Autodesk Fusion 360 part; units mm, degrees
(part 3 of 5)
  spline S32 degree 5 poles (-178.9509, -27.9451) (-178.953, -27.9386) (-178.9574, -27.9258) (-178.9646, -27.9067) (-178.975, -27.8817) (-178.9895, -27.8509) (-179.005, -27.8206) (-179.021, -27.7904) (-179.0374, -27.7604) (-179.0541, -27.7304) (-179.0709, -27.7005) (-179.0881, -27.6708) (-179.1057, -27.6412) (-179.1237, -27.6118) (-179.1422, -27.5825) (-179.1612, -27.5535) (-179.1805, -27.5247) (-179.2001, -27.4959) (-179.22, -27.4673) (-179.2402, -27.4388) (-179.2607, -27.4105) (-179.2814, -27.3822) (-179.3023, -27.3541) (-179.3236, -27.3261) (-179.3452, -27.2982) (-179.367, -27.2705) (-179.3891, -27.2429) (-179.4115, -27.2154) (-179.4341, -27.188) (-179.457, -27.1608) (-179.48, -27.1336) (-179.5033, -27.1066) (-179.5269, -27.0797) (-179.5506, -27.0529) (-179.5746, -27.0263) (-179.5989, -26.9997) (-179.6233, -26.9733) (-179.648, -26.947) (-179.6728, -26.9208) (-179.6979, -26.8947) (-179.7232, -26.8687) (-179.7487, -26.8428) (-179.7744, -26.8171) (-179.8003, -26.7914) (-179.8264, -26.7659) (-179.8527, -26.7405) (-179.8792, -26.7152) (-179.9058, -26.69) (-179.9327, -26.6649) (-179.9598, -26.64) (-179.987, -26.6151) (-180.0144, -26.5904) (-180.0421, -26.5658) (-180.0699, -26.5412) (-180.0978, -26.5168) (-180.126, -26.4926) (-180.1543, -26.4684) (-180.1828, -26.4443) (-180.2115, -26.4204) (-180.2404, -26.3965) (-180.2694, -26.3728) (-180.2986, -26.3492) (-180.3279, -26.3257) (-180.3575, -26.3023) (-180.3872, -26.279) (-180.417, -26.2558) (-180.447, -26.2328) (-180.4772, -26.2099) (-180.5076, -26.187) (-180.5381, -26.1643) (-180.5687, -26.1417) (-180.5934, -26.1237) (-180.612, -26.1103) (-180.6244, -26.1014) (-180.6306, -26.0969) knots 0 0 0 0 0 0 0.01428571 0.02857143 0.04285714 0.05714286 0.07142857 0.08571429 0.1 0.11428571 0.12857143 0.14285714 0.15714286 0.17142857 0.18571429 0.2 0.21428571 0.22857143 0.24285714 0.25714286 0.27142857 0.28571429 0.3 0.31428571 0.32857143 0.34285714 0.35714286 0.37142857 0.38571429 0.4 0.41428571 0.42857143 0.44285714 0.45714286 0.47142857 0.48571429 0.5 0.51428571 0.52857143 0.54285714 0.55714286 0.57142857 0.58571429 0.6 0.61428571 0.62857143 0.64285714 0.65714286 0.67142857 0.68571429 0.7 0.71428571 0.72857143 0.74285714 0.75714286 0.77142857 0.78571429 0.8 0.81428571 0.82857143 0.84285714 0.85714286 0.87142857 0.88571429 0.9 0.91428571 0.92857143 0.94285714 0.95714286 0.97142857 0.98571429 1 1 1 1 1 1
  arc A65 (-180.6306, -26.0969) -> (-181.4895, -26.4764) centre (-175, -40) ccw
  spline S33 degree 5 poles (-181.2537, -28.9627) (-181.2571, -28.9568) (-181.2636, -28.9449) (-181.2729, -28.9268) (-181.2843, -28.9022) (-181.2973, -28.8708) (-181.3094, -28.8389) (-181.3209, -28.8067) (-181.332, -28.7744) (-181.343, -28.7419) (-181.3537, -28.7093) (-181.3642, -28.6766) (-181.3743, -28.6437) (-181.3839, -28.6105) (-181.393, -28.5772) (-181.4017, -28.5436) (-181.41, -28.5099) (-181.418, -28.476) (-181.4258, -28.4421) (-181.4333, -28.408) (-181.4405, -28.3737) (-181.4474, -28.3394) (-181.4541, -28.305) (-181.4605, -28.2704) (-181.4666, -28.2357) (-181.4724, -28.2008) (-181.4779, -28.1659) (-181.4832, -28.1309) (-181.4882, -28.0957) (-181.493, -28.0605) (-181.4975, -28.0252) (-181.5018, -27.9897) (-181.5058, -27.9542) (-181.5096, -27.9186) (-181.5132, -27.8829) (-181.5165, -27.8471) (-181.5196, -27.8113) (-181.5225, -27.7753) (-181.5251, -27.7393) (-181.5275, -27.7032) (-181.5297, -27.667) (-181.5316, -27.6307) (-181.5334, -27.5944) (-181.5349, -27.558) (-181.5362, -27.5215) (-181.5373, -27.4849) (-181.5382, -27.4483) (-181.5388, -27.4116) (-181.5393, -27.3749) (-181.5395, -27.3381) (-181.5396, -27.3012) (-181.5394, -27.2643) (-181.539, -27.2273) (-181.5384, -27.1902) (-181.5376, -27.1531) (-181.5366, -27.1159) (-181.5354, -27.0787) (-181.534, -27.0414) (-181.5324, -27.0041) (-181.5306, -26.9667) (-181.5286, -26.9293) (-181.5264, -26.8918) (-181.524, -26.8542) (-181.5215, -26.8167) (-181.5187, -26.779) (-181.5157, -26.7414) (-181.5125, -26.7036) (-181.5092, -26.6659) (-181.5056, -26.6281) (-181.5019, -26.5902) (-181.4979, -26.5523) (-181.4947, -26.522) (-181.4921, -26.4992) (-181.4903, -26.484) (-181.4895, -26.4764) knots 0 0 0 0 0 0 0.01428571 0.02857143 0.04285714 0.05714286 0.07142857 0.08571429 0.1 0.11428571 0.12857143 0.14285714 0.15714286 0.17142857 0.18571429 0.2 0.21428571 0.22857143 0.24285714 0.25714286 0.27142857 0.28571429 0.3 0.31428571 0.32857143 0.34285714 0.35714286 0.37142857 0.38571429 0.4 0.41428571 0.42857143 0.44285714 0.45714286 0.47142857 0.48571429 0.5 0.51428571 0.52857143 0.54285714 0.55714286 0.57142857 0.58571429 0.6 0.61428571 0.62857143 0.64285714 0.65714286 0.67142857 0.68571429 0.7 0.71428571 0.72857143 0.74285714 0.75714286 0.77142857 0.78571429 0.8 0.81428571 0.82857143 0.84285714 0.85714286 0.87142857 0.88571429 0.9 0.91428571 0.92857143 0.94285714 0.95714286 0.97142857 0.98571429 1 1 1 1 1 1
  line L33 (-181.2537, -28.9627) -> (-181.041, -29.3382)
  arc A66 (-181.212, -30.0093) -> (-181.041, -29.3382) centre (-181.476, -29.5847) ccw
  arc A67 (-181.212, -30.0093) -> (-181.8833, -30.4594) centre (-175, -40) ccw
  arc A68 (-182.5691, -30.3628) -> (-181.8833, -30.4594) centre (-182.1759, -30.0539) ccw
  line L34 (-182.5691, -30.3628) -> (-182.8357, -30.0234)
  spline S34 degree 5 poles (-182.8357, -30.0234) (-182.8399, -30.018) (-182.8484, -30.0075) (-182.8616, -29.992) (-182.88, -29.9721) (-182.9041, -29.9481) (-182.9291, -29.9248) (-182.9545, -29.902) (-182.9801, -29.8794) (-183.006, -29.8569) (-183.0321, -29.8346) (-183.0584, -29.8125) (-183.085, -29.7907) (-183.112, -29.7692) (-183.1394, -29.7481) (-183.1671, -29.7273) (-183.1952, -29.7068) (-183.2235, -29.6866) (-183.252, -29.6665) (-183.2807, -29.6466) (-183.3096, -29.6269) (-183.3387, -29.6075) (-183.368, -29.5882) (-183.3976, -29.5692) (-183.4274, -29.5504) (-183.4574, -29.5318) (-183.4876, -29.5134) (-183.5181, -29.4952) (-183.5487, -29.4772) (-183.5794, -29.4594) (-183.6104, -29.4418) (-183.6415, -29.4244) (-183.6729, -29.4072) (-183.7044, -29.3901) (-183.736, -29.3733) (-183.7679, -29.3566) (-183.7999, -29.3401) (-183.8321, -29.3238) (-183.8644, -29.3077) (-183.8969, -29.2918) (-183.9295, -29.276) (-183.9623, -29.2604) (-183.9953, -29.245) (-184.0284, -29.2298) (-184.0616, -29.2147) (-184.095, -29.1999) (-184.1286, -29.1851) (-184.1623, -29.1706) (-184.1961, -29.1562) (-184.2301, -29.142) (-184.2642, -29.128) (-184.2984, -29.1141) (-184.3328, -29.1004) (-184.3673, -29.0869) (-184.4019, -29.0735) (-184.4367, -29.0603) (-184.4716, -29.0473) (-184.5066, -29.0345) (-184.5417, -29.0218) (-184.577, -29.0092) (-184.6124, -28.9969) (-184.6479, -28.9847) (-184.6835, -28.9726) (-184.7193, -28.9607) (-184.7551, -28.949) (-184.7911, -28.9375) (-184.8272, -28.9261) (-184.8634, -28.9148) (-184.8997, -28.9038) (-184.9362, -28.8928) (-184.9727, -28.8821) (-185.002, -28.8736) (-185.0241, -28.8673) (-185.0388, -28.8632) (-185.0462, -28.8611) knots 0 0 0 0 0 0 0.01428571 0.02857143 0.04285714 0.05714286 0.07142857 0.08571429 0.1 0.11428571 0.12857143 0.14285714 0.15714286 0.17142857 0.18571429 0.2 0.21428571 0.22857143 0.24285714 0.25714286 0.27142857 0.28571429 0.3 0.31428571 0.32857143 0.34285714 0.35714286 0.37142857 0.38571429 0.4 0.41428571 0.42857143 0.44285714 0.45714286 0.47142857 0.48571429 0.5 0.51428571 0.52857143 0.54285714 0.55714286 0.57142857 0.58571429 0.6 0.61428571 0.62857143 0.64285714 0.65714286 0.67142857 0.68571429 0.7 0.71428571 0.72857143 0.74285714 0.75714286 0.77142857 0.78571429 0.8 0.81428571 0.82857143 0.84285714 0.85714286 0.87142857 0.88571429 0.9 0.91428571 0.92857143 0.94285714 0.95714286 0.97142857 0.98571429 1 1 1 1 1 1
  arc A69 (-185.0462, -28.8611) -> (-185.7234, -29.5115) centre (-175, -40) ccw
  spline S35 degree 5 poles (-184.6515, -31.7672) (-184.6567, -31.7628) (-184.6669, -31.7539) (-184.6818, -31.74) (-184.701, -31.7208) (-184.724, -31.6958) (-184.7462, -31.6699) (-184.768, -31.6436) (-184.7896, -31.617) (-184.811, -31.5903) (-184.8322, -31.5633) (-184.8532, -31.5362) (-184.8739, -31.5087) (-184.8943, -31.4808) (-184.9143, -31.4526) (-184.9339, -31.424) (-184.9533, -31.3952) (-184.9724, -31.3661) (-184.9913, -31.3368) (-185.01, -31.3073) (-185.0285, -31.2777) (-185.0468, -31.2478) (-185.0648, -31.2177) (-185.0826, -31.1874) (-185.1002, -31.1568) (-185.1176, -31.1261) (-185.1347, -31.0952) (-185.1517, -31.064) (-185.1684, -31.0327) (-185.1849, -31.0013) (-185.2013, -30.9696) (-185.2174, -30.9378) (-185.2334, -30.9058) (-185.2491, -30.8736) (-185.2647, -30.8413) (-185.28, -30.8088) (-185.2952, -30.7762) (-185.3102, -30.7434) (-185.325, -30.7104) (-185.3396, -30.6773) (-185.354, -30.644) (-185.3683, -30.6106) (-185.3823, -30.5771) (-185.3962, -30.5434) (-185.4099, -30.5096) (-185.4235, -30.4756) (-185.4368, -30.4415) (-185.45, -30.4072) (-185.463, -30.3728) (-185.4758, -30.3383) (-185.4884, -30.3037) (-185.5009, -30.2689) (-185.5132, -30.234) (-185.5253, -30.199) (-185.5372, -30.1639) (-185.549, -30.1286) (-185.5606, -30.0932) (-185.5721, -30.0577) (-185.5833, -30.0221) (-185.5944, -29.9863) (-185.6054, -29.9505) (-185.6161, -29.9145) (-185.6267, -29.8784) (-185.6371, -29.8422) (-185.6474, -29.8059) (-185.6575, -29.7695) (-185.6674, -29.7329) (-185.6772, -29.6963) (-185.6868, -29.6596) (-185.6962, -29.6227) (-185.7054, -29.5858) (-185.7127, -29.5561) (-185.7181, -29.5338) (-185.7217, -29.519) (-185.7234, -29.5115) knots 0 0 0 0 0 0 0.01428571 0.02857143 0.04285714 0.05714286 0.07142857 0.08571429 0.1 0.11428571 0.12857143 0.14285714 0.15714286 0.17142857 0.18571429 0.2 0.21428571 0.22857143 0.24285714 0.25714286 0.27142857 0.28571429 0.3 0.31428571 0.32857143 0.34285714 0.35714286 0.37142857 0.38571429 0.4 0.41428571 0.42857143 0.44285714 0.45714286 0.47142857 0.48571429 0.5 0.51428571 0.52857143 0.54285714 0.55714286 0.57142857 0.58571429 0.6 0.61428571 0.62857143 0.64285714 0.65714286 0.67142857 0.68571429 0.7 0.71428571 0.72857143 0.74285714 0.75714286 0.77142857 0.78571429 0.8 0.81428571 0.82857143 0.84285714 0.85714286 0.87142857 0.88571429 0.9 0.91428571 0.92857143 0.94285714 0.95714286 0.97142857 0.98571429 1 1 1 1 1 1
  line L35 (-184.6515, -31.7672) -> (-184.3232, -32.0473)
  arc A70 (-184.2544, -32.7364) -> (-184.3232, -32.0473) centre (-184.6477, -32.4277) ccw
  arc A71 (-184.2544, -32.7364) -> (-184.7313, -33.389) centre (-175, -40) ccw
  circle A72 centre (-175, -40) radius 4
  line L36 (250, 25) -> (120, 25)
  line L37 (120, 25) -> (120, 175)
  line L38 (120, 175) -> (250, 175)
  line L39 (250, 175) -> (250, 25)
  dimension "d74" = 130
  dimension "d75" = 150
  constraint horizontal L36
  constraint vertical L37
  constraint horizontal L38
  constraint vertical L39
  measures "d74" distance of L36.start L36.end
  measures "d75" distance of L36.start L38.end
extrude "Extrude4" add sketch "SamsungFold4DeschisHusa" along normal blind 10 separate body contours L36 L37 L38 L39 makes body 5
sketch "Sketch6" plane through (0, 10, 0) normal (0, 1, 0) x (-1, 0, 0)
  arc A0 (-122.7744, -52.0505) -> (-123.3367, -51.6463) centre (-123.266, -52.1413) ccw
  line L0 (-122.7744, -52.0505) -> (-122.696, -52.4749)
  spline S0 degree 5 poles (-122.696, -52.4749) (-122.6947, -52.4815) (-122.6921, -52.4949) (-122.6876, -52.5147) (-122.6805, -52.5409) (-122.6703, -52.5733) (-122.6591, -52.6055) (-122.6472, -52.6375) (-122.6349, -52.6695) (-122.6225, -52.7014) (-122.6097, -52.7333) (-122.5967, -52.7651) (-122.5833, -52.7967) (-122.5693, -52.8283) (-122.5549, -52.8597) (-122.54, -52.891) (-122.5247, -52.9222) (-122.509, -52.9533) (-122.4931, -52.9843) (-122.4769, -53.0152) (-122.4605, -53.0461) (-122.4437, -53.0769) (-122.4267, -53.1076) (-122.4094, -53.1381) (-122.3917, -53.1686) (-122.3738, -53.199) (-122.3555, -53.2293) (-122.3371, -53.2596) (-122.3183, -53.2897) (-122.2993, -53.3198) (-122.2801, -53.3498) (-122.2606, -53.3797) (-122.2409, -53.4095) (-122.2209, -53.4392) (-122.2007, -53.4688) (-122.1802, -53.4984) (-122.1595, -53.5278) (-122.1386, -53.5572) (-122.1175, -53.5865) (-122.0961, -53.6157) (-122.0745, -53.6448) (-122.0527, -53.6739) (-122.0307, -53.7028) (-122.0085, -53.7317) (-121.986, -53.7605) (-121.9633, -53.7892) (-121.9405, -53.8178) (-121.9174, -53.8463) (-121.8941, -53.8748) (-121.8706, -53.9031) (-121.847, -53.9314) (-121.8231, -53.9596) (-121.799, -53.9877) (-121.7747, -54.0157) (-121.7503, -54.0436) (-121.7256, -54.0714) (-121.7008, -54.0992) (-121.6757, -54.1268) (-121.6505, -54.1544) (-121.6251, -54.1819) (-121.5995, -54.2093) (-121.5737, -54.2366) (-121.5478, -54.2638) (-121.5216, -54.2909) (-121.4953, -54.318) (-121.4688, -54.3449) (-121.4422, -54.3718) (-121.4153, -54.3985) (-121.3883, -54.4252) (-121.3611, -54.4518) (-121.3337, -54.4783) (-121.3117, -54.4994) (-121.2951, -54.5152) (-121.284, -54.5257) (-121.2784, -54.531) knots 0 0 0 0 0 0 0.01428571 0.02857143 0.04285714 0.05714286 0.07142857 0.08571429 0.1 0.11428571 0.12857143 0.14285714 0.15714286 0.17142857 0.18571429 0.2 0.21428571 0.22857143 0.24285714 0.25714286 0.27142857 0.28571429 0.3 0.31428571 0.32857143 0.34285714 0.35714286 0.37142857 0.38571429 0.4 0.41428571 0.42857143 0.44285714 0.45714286 0.47142857 0.48571429 0.5 0.51428571 0.52857143 0.54285714 0.55714286 0.57142857 0.58571429 0.6 0.61428571 0.62857143 0.64285714 0.65714286 0.67142857 0.68571429 0.7 0.71428571 0.72857143 0.74285714 0.75714286 0.77142857 0.78571429 0.8 0.81428571 0.82857143 0.84285714 0.85714286 0.87142857 0.88571429 0.9 0.91428571 0.92857143 0.94285714 0.95714286 0.97142857 0.98571429 1 1 1 1 1 1
  arc A1 (-121.2784, -54.531) -> (-120.3765, -54.2697) centre (-125, -40) ccw
  spline S1 degree 5 poles (-120.2778, -51.7742) (-120.2753, -51.7805) (-120.2704, -51.7932) (-120.2636, -51.8124) (-120.2556, -51.8383) (-120.2469, -51.8711) (-120.2392, -51.9043) (-120.2321, -51.9378) (-120.2254, -51.9713) (-120.2188, -52.005) (-120.2126, -52.0387) (-120.2066, -52.0725) (-120.201, -52.1065) (-120.1959, -52.1406) (-120.1913, -52.1749) (-120.1872, -52.2093) (-120.1834, -52.2438) (-120.18, -52.2785) (-120.1769, -52.3132) (-120.174, -52.348) (-120.1714, -52.3828) (-120.1691, -52.4178) (-120.1671, -52.4528) (-120.1654, -52.488) (-120.1641, -52.5232) (-120.163, -52.5585) (-120.1622, -52.5938) (-120.1616, -52.6292) (-120.1613, -52.6647) (-120.1613, -52.7003) (-120.1616, -52.7359) (-120.162, -52.7716) (-120.1628, -52.8073) (-120.1638, -52.8431) (-120.165, -52.879) (-120.1665, -52.9149) (-120.1682, -52.9508) (-120.1702, -52.9869) (-120.1724, -53.0229) (-120.1749, -53.059) (-120.1775, -53.0952) (-120.1804, -53.1314) (-120.1836, -53.1676) (-120.1869, -53.2039) (-120.1905, -53.2402) (-120.1943, -53.2766) (-120.1983, -53.313) (-120.2026, -53.3495) (-120.2071, -53.3859) (-120.2117, -53.4224) (-120.2166, -53.459) (-120.2218, -53.4956) (-120.2271, -53.5322) (-120.2326, -53.5688) (-120.2384, -53.6055) (-120.2443, -53.6422) (-120.2505, -53.679) (-120.2569, -53.7157) (-120.2634, -53.7525) (-120.2702, -53.7893) (-120.2772, -53.8261) (-120.2844, -53.863) (-120.2918, -53.8999) (-120.2993, -53.9368) (-120.3071, -53.9737) (-120.3151, -54.0106) (-120.3233, -54.0476) (-120.3317, -54.0846) (-120.3402, -54.1215) (-120.349, -54.1586) (-120.358, -54.1956) (-120.3653, -54.2252) (-120.3709, -54.2474) (-120.3746, -54.2623) (-120.3765, -54.2697) knots 0 0 0 0 0 0 0.01428571 0.02857143 0.04285714 0.05714286 0.07142857 0.08571429 0.1 0.11428571 0.12857143 0.14285714 0.15714286 0.17142857 0.18571429 0.2 0.21428571 0.22857143 0.24285714 0.25714286 0.27142857 0.28571429 0.3 0.31428571 0.32857143 0.34285714 0.35714286 0.37142857 0.38571429 0.4 0.41428571 0.42857143 0.44285714 0.45714286 0.47142857 0.48571429 0.5 0.51428571 0.52857143 0.54285714 0.55714286 0.57142857 0.58571429 0.6 0.61428571 0.62857143 0.64285714 0.65714286 0.67142857 0.68571429 0.7 0.71428571 0.72857143 0.74285714 0.75714286 0.77142857 0.78571429 0.8 0.81428571 0.82857143 0.84285714 0.85714286 0.87142857 0.88571429 0.9 0.91428571 0.92857143 0.94285714 0.95714286 0.97142857 0.98571429 1 1 1 1 1 1
  line L1 (-120.2778, -51.7742) -> (-120.4385, -51.3737)
  arc A2 (-120.1793, -50.7315) -> (-120.4385, -51.3737) centre (-119.9744, -51.1875) ccw
  arc A3 (-120.1793, -50.7315) -> (-119.4538, -50.3751) centre (-125, -40) ccw
  arc A4 (-118.7871, -50.5625) -> (-119.4538, -50.3751) centre (-119.218, -50.816) ccw
  line L2 (-118.7871, -50.5625) -> (-118.5683, -50.9345)
  spline S2 degree 5 poles (-118.5683, -50.9345) (-118.5648, -50.9404) (-118.5578, -50.952) (-118.5468, -50.9691) (-118.5312, -50.9913) (-118.5105, -51.0183) (-118.4889, -51.0446) (-118.4668, -51.0707) (-118.4443, -51.0965) (-118.4217, -51.1223) (-118.3989, -51.1478) (-118.3757, -51.1733) (-118.3523, -51.1984) (-118.3284, -51.2233) (-118.304, -51.2479) (-118.2793, -51.2722) (-118.2543, -51.2963) (-118.229, -51.3202) (-118.2034, -51.3439) (-118.1776, -51.3674) (-118.1516, -51.3908) (-118.1254, -51.4139) (-118.0989, -51.437) (-118.0721, -51.4598) (-118.0451, -51.4824) (-118.0178, -51.5048) (-117.9903, -51.5271) (-117.9626, -51.5491) (-117.9347, -51.5711) (-117.9066, -51.5928) (-117.8782, -51.6144) (-117.8497, -51.6358) (-117.821, -51.6571) (-117.792, -51.6782) (-117.7629, -51.6991) (-117.7336, -51.7199) (-117.704, -51.7405) (-117.6743, -51.761) (-117.6445, -51.7813) (-117.6144, -51.8014) (-117.5841, -51.8214) (-117.5537, -51.8412) (-117.5231, -51.8609) (-117.4923, -51.8804) (-117.4614, -51.8998) (-117.4303, -51.919) (-117.399, -51.9381) (-117.3676, -51.957) (-117.336, -51.9757) (-117.3042, -51.9944) (-117.2723, -52.0128) (-117.2402, -52.0311) (-117.208, -52.0493) (-117.1756, -52.0673) (-117.1431, -52.0852) (-117.1104, -52.1029) (-117.0775, -52.1205) (-117.0446, -52.1379) (-117.0114, -52.1552) (-116.9781, -52.1723) (-116.9447, -52.1893) (-116.9112, -52.2062) (-116.8775, -52.2229) (-116.8436, -52.2394) (-116.8096, -52.2558) (-116.7755, -52.2721) (-116.7413, -52.2882) (-116.7069, -52.3042) (-116.6724, -52.32) (-116.6377, -52.3357) (-116.603, -52.3512) (-116.575, -52.3635) (-116.554, -52.3727) (-116.54, -52.3788) (-116.533, -52.3818) knots 0 0 0 0 0 0 0.01428571 0.02857143 0.04285714 0.05714286 0.07142857 0.08571429 0.1 0.11428571 0.12857143 0.14285714 0.15714286 0.17142857 0.18571429 0.2 0.21428571 0.22857143 0.24285714 0.25714286 0.27142857 0.28571429 0.3 0.31428571 0.32857143 0.34285714 0.35714286 0.37142857 0.38571429 0.4 0.41428571 0.42857143 0.44285714 0.45714286 0.47142857 0.48571429 0.5 0.51428571 0.52857143 0.54285714 0.55714286 0.57142857 0.58571429 0.6 0.61428571 0.62857143 0.64285714 0.65714286 0.67142857 0.68571429 0.7 0.71428571 0.72857143 0.74285714 0.75714286 0.77142857 0.78571429 0.8 0.81428571 0.82857143 0.84285714 0.85714286 0.87142857 0.88571429 0.9 0.91428571 0.92857143 0.94285714 0.95714286 0.97142857 0.98571429 1 1 1 1 1 1
  arc A5 (-116.533, -52.3818) -> (-115.7748, -51.8278) centre (-125, -40) ccw
  spline S3 degree 5 poles (-116.5356, -49.4491) (-116.5311, -49.4541) (-116.5221, -49.4643) (-116.5092, -49.48) (-116.4928, -49.5016) (-116.4734, -49.5296) (-116.4548, -49.5581) (-116.4367, -49.5871) (-116.4189, -49.6163) (-116.4012, -49.6457) (-116.3838, -49.6753) (-116.3666, -49.705) (-116.3498, -49.735) (-116.3333, -49.7653) (-116.3173, -49.796) (-116.3016, -49.8269) (-116.2863, -49.8581) (-116.2712, -49.8894) (-116.2564, -49.921) (-116.2418, -49.9527) (-116.2275, -49.9846) (-116.2133, -50.0167) (-116.1995, -50.0489) (-116.1859, -50.0813) (-116.1725, -50.1139) (-116.1594, -50.1467) (-116.1466, -50.1797) (-116.134, -50.2128) (-116.1216, -50.246) (-116.1094, -50.2794) (-116.0974, -50.313) (-116.0857, -50.3467) (-116.0741, -50.3805) (-116.0628, -50.4145) (-116.0517, -50.4486) (-116.0408, -50.4829) (-116.0302, -50.5173) (-116.0197, -50.5518) (-116.0095, -50.5864) (-115.9994, -50.6212) (-115.9895, -50.6561) (-115.9799, -50.6911) (-115.9704, -50.7262) (-115.9612, -50.7614) (-115.9521, -50.7968) (-115.9433, -50.8323) (-115.9346, -50.8679) (-115.9261, -50.9036) (-115.9178, -50.9394) (-115.9098, -50.9753) (-115.9019, -51.0113) (-115.8942, -51.0474) (-115.8866, -51.0837) (-115.8793, -51.12) (-115.8722, -51.1564) (-115.8652, -51.193) (-115.8584, -51.2296) (-115.8518, -51.2663) (-115.8454, -51.3031) (-115.8392, -51.34) (-115.8332, -51.377) (-115.8273, -51.4141) (-115.8217, -51.4513) (-115.8162, -51.4886) (-115.8109, -51.5259) (-115.8057, -51.5634) (-115.8008, -51.6009) (-115.796, -51.6385) (-115.7914, -51.6762) (-115.787, -51.714) (-115.7827, -51.7518) (-115.7795, -51.7822) (-115.7771, -51.805) (-115.7756, -51.8202) (-115.7748, -51.8278) knots 0 0 0 0 0 0 0.01428571 0.02857143 0.04285714 0.05714286 0.07142857 0.08571429 0.1 0.11428571 0.12857143 0.14285714 0.15714286 0.17142857 0.18571429 0.2 0.21428571 0.22857143 0.24285714 0.25714286 0.27142857 0.28571429 0.3 0.31428571 0.32857143 0.34285714 0.35714286 0.37142857 0.38571429 0.4 0.41428571 0.42857143 0.44285714 0.45714286 0.47142857 0.48571429 0.5 0.51428571 0.52857143 0.54285714 0.55714286 0.57142857 0.58571429 0.6 0.61428571 0.62857143 0.64285714 0.65714286 0.67142857 0.68571429 0.7 0.71428571 0.72857143 0.74285714 0.75714286 0.77142857 0.78571429 0.8 0.81428571 0.82857143 0.84285714 0.85714286 0.87142857 0.88571429 0.9 0.91428571 0.92857143 0.94285714 0.95714286 0.97142857 0.98571429 1 1 1 1 1 1
  line L3 (-116.5356, -49.4491) -> (-116.8235, -49.1276)
  arc A6 (-116.7996, -48.4355) -> (-116.8235, -49.1276) centre (-116.4511, -48.794) ccw
  arc A7 (-116.7996, -48.4355) -> (-116.2397, -47.8525) centre (-125, -40) ccw
  arc A8 (-115.5491, -47.8006) -> (-116.2397, -47.8525) centre (-115.8674, -48.1862) ccw
  line L4 (-115.5491, -47.8006) -> (-115.2163, -48.0753)
  spline S4 degree 5 poles (-115.2163, -48.0753) (-115.2111, -48.0796) (-115.2005, -48.0881) (-115.1843, -48.1004) (-115.162, -48.116) (-115.1334, -48.1342) (-115.1041, -48.1516) (-115.0744, -48.1685) (-115.0445, -48.1852) (-115.0144, -48.2016) (-114.9842, -48.2178) (-114.9537, -48.2338) (-114.9231, -48.2494) (-114.8921, -48.2646) (-114.8609, -48.2794) (-114.8293, -48.2938) (-114.7976, -48.3079) (-114.7656, -48.3216) (-114.7335, -48.3352) (-114.7012, -48.3485) (-114.6687, -48.3615) (-114.6361, -48.3743) (-114.6034, -48.3869) (-114.5704, -48.3992) (-114.5373, -48.4112) (-114.504, -48.4229) (-114.4706, -48.4344) (-114.437, -48.4457) (-114.4032, -48.4568) (-114.3694, -48.4676) (-114.3354, -48.4782) (-114.3012, -48.4886) (-114.267, -48.4987) (-114.2325, -48.5086) (-114.198, -48.5183) (-114.1633, -48.5278) (-114.1286, -48.5371) (-114.0936, -48.5462) (-114.0586, -48.555) (-114.0235, -48.5637) (-113.9882, -48.5721) (-113.9528, -48.5803) (-113.9174, -48.5883) (-113.8818, -48.5962) (-113.8461, -48.6038) (-113.8103, -48.6112) (-113.7744, -48.6184) (-113.7383, -48.6254) (-113.7022, -48.6323) (-113.666, -48.6389) (-113.6297, -48.6453) (-113.5933, -48.6516) (-113.5568, -48.6576) (-113.5202, -48.6635) (-113.4835, -48.6691) (-113.4467, -48.6746) (-113.4099, -48.6799) (-113.3729, -48.685) (-113.3359, -48.6899) (-113.2987, -48.6946) (-113.2615, -48.6992) (-113.2242, -48.7035) (-113.1869, -48.7077) (-113.1494, -48.7116) (-113.1119, -48.7154) (-113.0742, -48.7191) (-113.0365, -48.7225) (-112.9988, -48.7257) (-112.9609, -48.7288) (-112.923, -48.7317) (-112.885, -48.7344) (-112.8545, -48.7364) (-112.8317, -48.7378) (-112.8164, -48.7388) (-112.8088, -48.7392) knots 0 0 0 0 0 0 0.01428571 0.02857143 0.04285714 0.05714286 0.07142857 0.08571429 0.1 0.11428571 0.12857143 0.14285714 0.15714286 0.17142857 0.18571429 0.2 0.21428571 0.22857143 0.24285714 0.25714286 0.27142857 0.28571429 0.3 0.31428571 0.32857143 0.34285714 0.35714286 0.37142857 0.38571429 0.4 0.41428571 0.42857143 0.44285714 0.45714286 0.47142857 0.48571429 0.5 0.51428571 0.52857143 0.54285714 0.55714286 0.57142857 0.58571429 0.6 0.61428571 0.62857143 0.64285714 0.65714286 0.67142857 0.68571429 0.7 0.71428571 0.72857143 0.74285714 0.75714286 0.77142857 0.78571429 0.8 0.81428571 0.82857143 0.84285714 0.85714286 0.87142857 0.88571429 0.9 0.91428571 0.92857143 0.94285714 0.95714286 0.97142857 0.98571429 1 1 1 1 1 1
  arc A9 (-112.8088, -48.7392) -> (-112.2858, -47.9593) centre (-125, -40) ccw
  spline S5 degree 5 poles (-113.8143, -45.9842) (-113.8083, -45.9874) (-113.7964, -45.994) (-113.7789, -46.0043) (-113.7561, -46.019) (-113.7283, -46.0386) (-113.701, -46.0591) (-113.6741, -46.0801) (-113.6474, -46.1015) (-113.6208, -46.1231) (-113.5943, -46.1449) (-113.568, -46.1669) (-113.5419, -46.1894) (-113.516, -46.2122) (-113.4905, -46.2355) (-113.4652, -46.2592) (-113.4401, -46.2833) (-113.4152, -46.3076) (-113.3905, -46.3322) (-113.366, -46.357) (-113.3416, -46.3821) (-113.3173, -46.4074) (-113.2933, -46.4329) (-113.2694, -46.4587) (-113.2457, -46.4848) (-113.2222, -46.5111) (-113.1989, -46.5377) (-113.1757, -46.5645) (-113.1526, -46.5915) (-113.1298, -46.6187) (-113.1071, -46.6462) (-113.0845, -46.6738) (-113.0621, -46.7017) (-113.0398, -46.7297) (-113.0177, -46.758) (-112.9958, -46.7865) (-112.974, -46.8151) (-112.9524, -46.844) (-112.9309, -46.873) (-112.9095, -46.9023) (-112.8884, -46.9317) (-112.8673, -46.9613) (-112.8464, -46.991) (-112.8257, -47.021) (-112.8051, -47.0511) (-112.7846, -47.0814) (-112.7643, -47.1119) (-112.7441, -47.1426) (-112.7241, -47.1734) (-112.7042, -47.2044) (-112.6845, -47.2355) (-112.6649, -47.2668) (-112.6454, -47.2983) (-112.6261, -47.3299) (-112.6069, -47.3617) (-112.5879, -47.3937) (-112.569, -47.4258) (-112.5502, -47.458) (-112.5316, -47.4904) (-112.5132, -47.523) (-112.4948, -47.5557) (-112.4767, -47.5885) (-112.4586, -47.6215) (-112.4407, -47.6547) (-112.4229, -47.6879) (-112.4053, -47.7214) (-112.3878, -47.7549) (-112.3705, -47.7887) (-112.3533, -47.8225) (-112.3362, -47.8565) (-112.3193, -47.8906) (-112.3058, -47.918) (-112.2958, -47.9386) (-112.2892, -47.9524) (-112.2858, -47.9593) knots 0 0 0 0 0 0 0.01428571 0.02857143 0.04285714 0.05714286 0.07142857 0.08571429 0.1 0.11428571 0.12857143 0.14285714 0.15714286 0.17142857 0.18571429 0.2 0.21428571 0.22857143 0.24285714 0.25714286 0.27142857 0.28571429 0.3 0.31428571 0.32857143 0.34285714 0.35714286 0.37142857 0.38571429 0.4 0.41428571 0.42857143 0.44285714 0.45714286 0.47142857 0.48571429 0.5 0.51428571 0.52857143 0.54285714 0.55714286 0.57142857 0.58571429 0.6 0.61428571 0.62857143 0.64285714 0.65714286 0.67142857 0.68571429 0.7 0.71428571 0.72857143 0.74285714 0.75714286 0.77142857 0.78571429 0.8 0.81428571 0.82857143 0.84285714 0.85714286 0.87142857 0.88571429 0.9 0.91428571 0.92857143 0.94285714 0.95714286 0.97142857 0.98571429 1 1 1 1 1 1
  line L5 (-113.8143, -45.9842) -> (-114.1948, -45.7806)
  arc A10 (-114.4091, -45.1221) -> (-114.1948, -45.7806) centre (-113.9589, -45.3398) ccw
  arc A11 (-114.4091, -45.1221) -> (-114.0823, -44.3827) centre (-125, -40) ccw
  arc A12 (-113.4511, -44.0978) -> (-114.0823, -44.3827) centre (-113.6183, -44.569) ccw
  line L6 (-113.4511, -44.0978) -> (-113.0444, -44.2421)
  spline S6 degree 5 poles (-113.0444, -44.2421) (-113.038, -44.2444) (-113.0252, -44.2487) (-113.0057, -44.2547) (-112.9795, -44.2617) (-112.9463, -44.2691) (-112.9128, -44.2754) (-112.8792, -44.2812) (-112.8454, -44.2865) (-112.8115, -44.2917) (-112.7775, -44.2966) (-112.7435, -44.3012) (-112.7093, -44.3054) (-112.675, -44.3091) (-112.6406, -44.3123) (-112.606, -44.3151) (-112.5714, -44.3174) (-112.5366, -44.3194) (-112.5018, -44.3211) (-112.4669, -44.3226) (-112.432, -44.3238) (-112.397, -44.3247) (-112.3619, -44.3252) (-112.3267, -44.3255) (-112.2915, -44.3255) (-112.2562, -44.3251) (-112.2208, -44.3245) (-112.1854, -44.3236) (-112.1499, -44.3225) (-112.1144, -44.321) (-112.0788, -44.3194) (-112.0432, -44.3174) (-112.0075, -44.3153) (-111.9718, -44.3128) (-111.936, -44.3101) (-111.9002, -44.3072) (-111.8643, -44.304) (-111.8284, -44.3006) (-111.7925, -44.2969) (-111.7565, -44.293) (-111.7205, -44.2889) (-111.6844, -44.2845) (-111.6483, -44.2799) (-111.6122, -44.2751) (-111.5761, -44.27) (-111.5399, -44.2648) (-111.5037, -44.2593) (-111.4674, -44.2535) (-111.4312, -44.2476) (-111.3949, -44.2415) (-111.3585, -44.2351) (-111.3222, -44.2285) (-111.2858, -44.2217) (-111.2494, -44.2147) (-111.213, -44.2075) (-111.1766, -44.2) (-111.1401, -44.1924) (-111.1037, -44.1845) (-111.0672, -44.1765) (-111.0307, -44.1682) (-110.9942, -44.1597) (-110.9576, -44.1511) (-110.9211, -44.1422) (-110.8845, -44.1331) (-110.8479, -44.1238) (-110.8114, -44.1144) (-110.7748, -44.1047) (-110.7382, -44.0948) (-110.7015, -44.0848) (-110.6649, -44.0745) (-110.6283, -44.0641) (-110.599, -44.0556) (-110.577, -44.0491) (-110.5623, -44.0447) (-110.555, -44.0425) knots 0 0 0 0 0 0 0.01428571 0.02857143 0.04285714 0.05714286 0.07142857 0.08571429 0.1 0.11428571 0.12857143 0.14285714 0.15714286 0.17142857 0.18571429 0.2 0.21428571 0.22857143 0.24285714 0.25714286 0.27142857 0.28571429 0.3 0.31428571 0.32857143 0.34285714 0.35714286 0.37142857 0.38571429 0.4 0.41428571 0.42857143 0.44285714 0.45714286 0.47142857 0.48571429 0.5 0.51428571 0.52857143 0.54285714 0.55714286 0.57142857 0.58571429 0.6 0.61428571 0.62857143 0.64285714 0.65714286 0.67142857 0.68571429 0.7 0.71428571 0.72857143 0.74285714 0.75714286 0.77142857 0.78571429 0.8 0.81428571 0.82857143 0.84285714 0.85714286 0.87142857 0.88571429 0.9 0.91428571 0.92857143 0.94285714 0.95714286 0.97142857 0.98571429 1 1 1 1 1 1
  arc A13 (-110.555, -44.0425) -> (-110.3304, -43.1308) centre (-125, -40) ccw
  spline S7 degree 5 poles (-112.4422, -41.7976) (-112.4354, -41.7985) (-112.422, -41.8006) (-112.402, -41.8044) (-112.3755, -41.8103) (-112.3427, -41.8192) (-112.3101, -41.8292) (-112.2776, -41.8398) (-112.2452, -41.8507) (-112.2128, -41.8619) (-112.1805, -41.8733) (-112.1482, -41.885) (-112.116, -41.8972) (-112.0839, -41.9098) (-112.0519, -41.923) (-112.02, -41.9366) (-111.9883, -41.9506) (-111.9566, -41.965) (-111.9249, -41.9797) (-111.8934, -41.9946) (-111.8619, -42.0098) (-111.8304, -42.0253) (-111.7991, -42.041) (-111.7678, -42.0571) (-111.7366, -42.0735) (-111.7055, -42.0902) (-111.6745, -42.1072) (-111.6436, -42.1245) (-111.6127, -42.142) (-111.5819, -42.1597) (-111.5512, -42.1777) (-111.5205, -42.196) (-111.4899, -42.2145) (-111.4594, -42.2333) (-111.429, -42.2523) (-111.3986, -42.2715) (-111.3684, -42.291) (-111.3382, -42.3107) (-111.308, -42.3306) (-111.278, -42.3508) (-111.248, -42.3712) (-111.2181, -42.3918) (-111.1883, -42.4127) (-111.1585, -42.4337) (-111.1289, -42.455) (-111.0993, -42.4765) (-111.0698, -42.4981) (-111.0403, -42.52) (-111.011, -42.5422) (-110.9817, -42.5645) (-110.9525, -42.587) (-110.9234, -42.6097) (-110.8943, -42.6326) (-110.8653, -42.6557) (-110.8365, -42.6791) (-110.8077, -42.7026) (-110.7789, -42.7263) (-110.7503, -42.7502) (-110.7217, -42.7743) (-110.6932, -42.7985) (-110.6648, -42.823) (-110.6365, -42.8476) (-110.6082, -42.8725) (-110.5801, -42.8975) (-110.552, -42.9227) (-110.524, -42.9481) (-110.4961, -42.9736) (-110.4683, -42.9994) (-110.4405, -43.0253) (-110.4128, -43.0514) (-110.3853, -43.0777) (-110.3633, -43.0988) (-110.3468, -43.1148) (-110.3358, -43.1254) (-110.3304, -43.1308) knots 0 0 0 0 0 0 0.01428571 0.02857143 0.04285714 0.05714286 0.07142857 0.08571429 0.1 0.11428571 0.12857143 0.14285714 0.15714286 0.17142857 0.18571429 0.2 0.21428571 0.22857143 0.24285714 0.25714286 0.27142857 0.28571429 0.3 0.31428571 0.32857143 0.34285714 0.35714286 0.37142857 0.38571429 0.4 0.41428571 0.42857143 0.44285714 0.45714286 0.47142857 0.48571429 0.5 0.51428571 0.52857143 0.54285714 0.55714286 0.57142857 0.58571429 0.6 0.61428571 0.62857143 0.64285714 0.65714286 0.67142857 0.68571429 0.7 0.71428571 0.72857143 0.74285714 0.75714286 0.77142857 0.78571429 0.8 0.81428571 0.82857143 0.84285714 0.85714286 0.87142857 0.88571429 0.9 0.91428571 0.92857143 0.94285714 0.95714286 0.97142857 0.98571429 1 1 1 1 1 1
  line L7 (-112.4422, -41.7976) -> (-112.8693, -41.7364)
  arc A14 (-113.2959, -41.1909) -> (-112.8693, -41.7364) centre (-112.7985, -41.2415) ccw
  arc A15 (-113.2959, -41.1909) -> (-113.2418, -40.3844) centre (-125, -40) ccw
  arc A16 (-112.7461, -39.9007) -> (-113.2418, -40.3844) centre (-112.742, -40.4007) ccw
  line L8 (-112.7461, -39.9007) -> (-112.3146, -39.8972)
  spline S8 degree 5 poles (-112.3146, -39.8972) (-112.3078, -39.8972) (-112.2942, -39.8969) (-112.2739, -39.8959) (-112.2468, -39.8935) (-112.2131, -39.889) (-112.1795, -39.8835) (-112.1459, -39.8774) (-112.1123, -39.8709) (-112.0787, -39.8642) (-112.0451, -39.8572) (-112.0115, -39.8498) (-111.978, -39.8421) (-111.9445, -39.8338) (-111.9111, -39.8251) (-111.8777, -39.8158) (-111.8443, -39.8062) (-111.8109, -39.7962) (-111.7776, -39.7859) (-111.7444, -39.7753) (-111.7111, -39.7645) (-111.6779, -39.7534) (-111.6447, -39.7419) (-111.6116, -39.7301) (-111.5785, -39.718) (-111.5454, -39.7057) (-111.5124, -39.693) (-111.4795, -39.68) (-111.4465, -39.6668) (-111.4136, -39.6533) (-111.3807, -39.6396) (-111.3479, -39.6256) (-111.3151, -39.6113) (-111.2824, -39.5968) (-111.2497, -39.582) (-111.2171, -39.567) (-111.1844, -39.5518) (-111.1519, -39.5363) (-111.1194, -39.5205) (-111.0869, -39.5046) (-111.0545, -39.4884) (-111.0221, -39.4719) (-110.9897, -39.4553) (-110.9574, -39.4384) (-110.9252, -39.4213) (-110.893, -39.4039) (-110.8608, -39.3864) (-110.8287, -39.3686) (-110.7967, -39.3506) (-110.7647, -39.3324) (-110.7327, -39.314) (-110.7008, -39.2954) (-110.669, -39.2766) (-110.6372, -39.2575) (-110.6055, -39.2383) (-110.5738, -39.2188) (-110.5421, -39.1992) (-110.5105, -39.1793) (-110.479, -39.1593) (-110.4475, -39.139) (-110.4161, -39.1186) (-110.3847, -39.0979) (-110.3534, -39.0771) (-110.3222, -39.0561) (-110.291, -39.0349) (-110.2598, -39.0134) (-110.2287, -38.9918) (-110.1977, -38.9701) (-110.1668, -38.9481) (-110.1359, -38.9259) (-110.105, -38.9036) (-110.0804, -38.8855) (-110.0619, -38.8719) (-110.0497, -38.8628) (-110.0435, -38.8583) knots 0 0 0 0 0 0 0.01428571 0.02857143 0.04285714 0.05714286 0.07142857 0.08571429 0.1 0.11428571 0.12857143 0.14285714 0.15714286 0.17142857 0.18571429 0.2 0.21428571 0.22857143 0.24285714 0.25714286 0.27142857 0.28571429 0.3 0.31428571 0.32857143 0.34285714 0.35714286 0.37142857 0.38571429 0.4 0.41428571 0.42857143 0.44285714 0.45714286 0.47142857 0.48571429 0.5 0.51428571 0.52857143 0.54285714 0.55714286 0.57142857 0.58571429 0.6 0.61428571 0.62857143 0.64285714 0.65714286 0.67142857 0.68571429 0.7 0.71428571 0.72857143 0.74285714 0.75714286 0.77142857 0.78571429 0.8 0.81428571 0.82857143 0.84285714 0.85714286 0.87142857 0.88571429 0.9 0.91428571 0.92857143 0.94285714 0.95714286 0.97142857 0.98571429 1 1 1 1 1 1
  arc A17 (-110.0435, -38.8583) -> (-110.1443, -37.9247) centre (-125, -40) ccw
  spline S9 degree 5 poles (-112.5847, -37.3941) (-112.578, -37.3927) (-112.5647, -37.3901) (-112.5446, -37.3868) (-112.5177, -37.3833) (-112.4838, -37.3805) (-112.4498, -37.3787) (-112.4157, -37.3775) (-112.3814, -37.3767) (-112.3472, -37.3761) (-112.3129, -37.3758) (-112.2785, -37.3758) (-112.2441, -37.3762) (-112.2096, -37.3771) (-112.1751, -37.3785) (-112.1405, -37.3804) (-112.1058, -37.3827) (-112.0711, -37.3854) (-112.0364, -37.3883) (-112.0016, -37.3916) (-111.9668, -37.3951) (-111.932, -37.3989) (-111.8971, -37.403) (-111.8622, -37.4074) (-111.8273, -37.4121) (-111.7924, -37.4172) (-111.7574, -37.4226) (-111.7224, -37.4282) (-111.6874, -37.4341) (-111.6524, -37.4402) (-111.6174, -37.4466) (-111.5823, -37.4533) (-111.5473, -37.4602) (-111.5122, -37.4674) (-111.4771, -37.4749) (-111.442, -37.4826) (-111.4069, -37.4905) (-111.3718, -37.4987) (-111.3366, -37.5072) (-111.3015, -37.5158) (-111.2664, -37.5247) (-111.2312, -37.5339) (-111.1961, -37.5433) (-111.1609, -37.5529) (-111.1258, -37.5627) (-111.0906, -37.5728) (-111.0554, -37.5831) (-111.0203, -37.5936) (-110.9851, -37.6043) (-110.95, -37.6153) (-110.9149, -37.6264) (-110.8797, -37.6378) (-110.8446, -37.6494) (-110.8095, -37.6612) (-110.7743, -37.6733) (-110.7392, -37.6855) (-110.7041, -37.698) (-110.669, -37.7106) (-110.6339, -37.7235) (-110.5989, -37.7365) (-110.5638, -37.7498) (-110.5288, -37.7633) (-110.4937, -37.777) (-110.4587, -37.7909) (-110.4237, -37.8049) (-110.3887, -37.8192) (-110.3537, -37.8337) (-110.3188, -37.8484) (-110.2838, -37.8632) (-110.2489, -37.8783) (-110.214, -37.8935) (-110.1861, -37.9059) (-110.1652, -37.9152) (-110.1512, -37.9215) (-110.1443, -37.9247) knots 0 0 0 0 0 0 0.01428571 0.02857143 0.04285714 0.05714286 0.07142857 0.08571429 0.1 0.11428571 0.12857143 0.14285714 0.15714286 0.17142857 0.18571429 0.2 0.21428571 0.22857143 0.24285714 0.25714286 0.27142857 0.28571429 0.3 0.31428571 0.32857143 0.34285714 0.35714286 0.37142857 0.38571429 0.4 0.41428571 0.42857143 0.44285714 0.45714286 0.47142857 0.48571429 0.5 0.51428571 0.52857143 0.54285714 0.55714286 0.57142857 0.58571429 0.6 0.61428571 0.62857143 0.64285714 0.65714286 0.67142857 0.68571429 0.7 0.71428571 0.72857143 0.74285714 0.75714286 0.77142857 0.78571429 0.8 0.81428571 0.82857143 0.84285714 0.85714286 0.87142857 0.88571429 0.9 0.91428571 0.92857143 0.94285714 0.95714286 0.97142857 0.98571429 1 1 1 1 1 1
  line L9 (-112.5847, -37.3941) -> (-113.007, -37.4828)
  arc A18 (-113.5945, -37.116) -> (-113.007, -37.4828) centre (-113.1097, -36.9934) ccw
  arc A19 (-113.5945, -37.116) -> (-113.8194, -36.3396) centre (-125, -40) ccw
  arc A20 (-113.5191, -35.7156) -> (-113.8194, -36.3396) centre (-113.3442, -36.1841) ccw
  line L10 (-113.5191, -35.7156) -> (-113.1147, -35.5647)
  spline S10 degree 5 poles (-113.1147, -35.5647) (-113.1084, -35.5624) (-113.0957, -35.5575) (-113.077, -35.5496) (-113.0524, -35.5381) (-113.0222, -35.5224) (-112.9925, -35.5057) (-112.963, -35.4884) (-112.9337, -35.4708) (-112.9044, -35.453) (-112.8752, -35.4349) (-112.8462, -35.4166) (-112.8173, -35.3978) (-112.7887, -35.3786) (-112.7602, -35.3589) (-112.732, -35.3388) (-112.704, -35.3184) (-112.676, -35.2976) (-112.6483, -35.2765) (-112.6206, -35.2552) (-112.5931, -35.2336) (-112.5657, -35.2118) (-112.5384, -35.1897) (-112.5113, -35.1673) (-112.4844, -35.1446) (-112.4575, -35.1217) (-112.4308, -35.0985) (-112.4043, -35.075) (-112.3778, -35.0513) (-112.3515, -35.0274) (-112.3254, -35.0032) (-112.2993, -34.9789) (-112.2734, -34.9543) (-112.2476, -34.9294) (-112.2219, -34.9044) (-112.1964, -34.8791) (-112.1709, -34.8536) (-112.1456, -34.8279) (-112.1205, -34.802) (-112.0954, -34.7759) (-112.0705, -34.7496) (-112.0457, -34.723) (-112.021, -34.6963) (-111.9964, -34.6694) (-111.9719, -34.6423) (-111.9476, -34.615) (-111.9234, -34.5875) (-111.8993, -34.5598) (-111.8754, -34.532) (-111.8515, -34.5039) (-111.8278, -34.4757) (-111.8042, -34.4473) (-111.7807, -34.4187) (-111.7573, -34.3899) (-111.7341, -34.361) (-111.7109, -34.3319) (-111.6879, -34.3026) (-111.665, -34.2731) (-111.6423, -34.2435) (-111.6196, -34.2137) (-111.5971, -34.1838) (-111.5747, -34.1536) (-111.5524, -34.1233) (-111.5302, -34.0929) (-111.5081, -34.0623) (-111.4862, -34.0315) (-111.4644, -34.0006) (-111.4427, -33.9695) (-111.4211, -33.9382) (-111.3996, -33.9069) (-111.3783, -33.8753) (-111.3613, -33.8499) (-111.3486, -33.8308) (-111.3402, -33.8181) (-111.336, -33.8117) knots 0 0 0 0 0 0 0.01428571 0.02857143 0.04285714 0.05714286 0.07142857 0.08571429 0.1 0.11428571 0.12857143 0.14285714 0.15714286 0.17142857 0.18571429 0.2 0.21428571 0.22857143 0.24285714 0.25714286 0.27142857 0.28571429 0.3 0.31428571 0.32857143 0.34285714 0.35714286 0.37142857 0.38571429 0.4 0.41428571 0.42857143 0.44285714 0.45714286 0.47142857 0.48571429 0.5 0.51428571 0.52857143 0.54285714 0.55714286 0.57142857 0.58571429 0.6 0.61428571 0.62857143 0.64285714 0.65714286 0.67142857 0.68571429 0.7 0.71428571 0.72857143 0.74285714 0.75714286 0.77142857 0.78571429 0.8 0.81428571 0.82857143 0.84285714 0.85714286 0.87142857 0.88571429 0.9 0.91428571 0.92857143 0.94285714 0.95714286 0.97142857 0.98571429 1 1 1 1 1 1
  arc A21 (-111.336, -33.8117) -> (-111.75, -32.9689) centre (-125, -40) ccw
  spline S11 degree 5 poles (-114.2247, -33.305) (-114.2189, -33.3014) (-114.2073, -33.2944) (-114.1896, -33.2844) (-114.1654, -33.272) (-114.1346, -33.2577) (-114.1032, -33.2443) (-114.0715, -33.2316) (-114.0397, -33.2191) (-114.0077, -33.2068) (-113.9755, -33.1948) (-113.9433, -33.183) (-113.9108, -33.1716) (-113.8781, -33.1607) (-113.8451, -33.1502) (-113.8119, -33.1402) (-113.7786, -33.1305) (-113.7451, -33.1211) (-113.7114, -33.112) (-113.6776, -33.1031) (-113.6437, -33.0945) (-113.6097, -33.0862) (-113.5756, -33.0781) (-113.5413, -33.0704) (-113.5068, -33.0629) (-113.4723, -33.0557) (-113.4376, -33.0488) (-113.4028, -33.0421) (-113.3679, -33.0356) (-113.3329, -33.0295) (-113.2978, -33.0235) (-113.2625, -33.0178) (-113.2272, -33.0123) (-113.1918, -33.0071) (-113.1563, -33.0021) (-113.1207, -32.9973) (-113.0849, -32.9927) (-113.0491, -32.9884) (-113.0132, -32.9844) (-112.9772, -32.9805) (-112.9412, -32.9768) (-112.905, -32.9734) (-112.8688, -32.9702) (-112.8325, -32.9672) (-112.7961, -32.9644) (-112.7596, -32.9619) (-112.723, -32.9595) (-112.6864, -32.9574) (-112.6497, -32.9554) (-112.6129, -32.9537) (-112.5761, -32.9522) (-112.5392, -32.9509) (-112.5022, -32.9497) (-112.4651, -32.9488) (-112.428, -32.9481) (-112.3909, -32.9476) (-112.3536, -32.9473) (-112.3163, -32.9472) (-112.2789, -32.9473) (-112.2415, -32.9476) (-112.204, -32.9481) (-112.1665, -32.9487) (-112.1289, -32.9496) (-112.0912, -32.9507) (-112.0535, -32.9519) (-112.0157, -32.9534) (-111.9779, -32.955) (-111.9401, -32.9568) (-111.9021, -32.9589) (-111.8642, -32.9611) (-111.8262, -32.9635) (-111.7957, -32.9655) (-111.7729, -32.9672) (-111.7576, -32.9683) (-111.75, -32.9689) knots 0 0 0 0 0 0 0.01428571 0.02857143 0.04285714 0.05714286 0.07142857 0.08571429 0.1 0.11428571 0.12857143 0.14285714 0.15714286 0.17142857 0.18571429 0.2 0.21428571 0.22857143 0.24285714 0.25714286 0.27142857 0.28571429 0.3 0.31428571 0.32857143 0.34285714 0.35714286 0.37142857 0.38571429 0.4 0.41428571 0.42857143 0.44285714 0.45714286 0.47142857 0.48571429 0.5 0.51428571 0.52857143 0.54285714 0.55714286 0.57142857 0.58571429 0.6 0.61428571 0.62857143 0.64285714 0.65714286 0.67142857 0.68571429 0.7 0.71428571 0.72857143 0.74285714 0.75714286 0.77142857 0.78571429 0.8 0.81428571 0.82857143 0.84285714 0.85714286 0.87142857 0.88571429 0.9 0.91428571 0.92857143 0.94285714 0.95714286 0.97142857 0.98571429 1 1 1 1 1 1
  line L11 (-114.2247, -33.305) -> (-114.5912, -33.5327)
  arc A22 (-115.2687, -33.389) -> (-114.5912, -33.5327) centre (-114.8551, -33.108) ccw
  arc A23 (-115.2687, -33.389) -> (-115.7456, -32.7364) centre (-125, -40) ccw
  arc A24 (-115.6768, -32.0473) -> (-115.7456, -32.7364) centre (-115.3523, -32.4277) ccw
  line L12 (-115.6768, -32.0473) -> (-115.3485, -31.7672)
  spline S12 degree 5 poles (-115.3485, -31.7672) (-115.3433, -31.7628) (-115.3331, -31.7539) (-115.3182, -31.74) (-115.299, -31.7208) (-115.276, -31.6958) (-115.2538, -31.6699) (-115.232, -31.6436) (-115.2104, -31.617) (-115.189, -31.5903) (-115.1678, -31.5633) (-115.1468, -31.5362) (-115.1261, -31.5087) (-115.1057, -31.4808) (-115.0857, -31.4526) (-115.0661, -31.424) (-115.0467, -31.3952) (-115.0276, -31.3661) (-115.0087, -31.3368) (-114.99, -31.3073) (-114.9715, -31.2777) (-114.9532, -31.2478) (-114.9352, -31.2177) (-114.9174, -31.1874) (-114.8998, -31.1568) (-114.8824, -31.1261) (-114.8653, -31.0952) (-114.8483, -31.064) (-114.8316, -31.0327) (-114.8151, -31.0013) (-114.7987, -30.9696) (-114.7826, -30.9378) (-114.7666, -30.9058) (-114.7509, -30.8736) (-114.7353, -30.8413) (-114.72, -30.8088) (-114.7048, -30.7762) (-114.6898, -30.7434) (-114.675, -30.7104) (-114.6604, -30.6773) (-114.646, -30.644) (-114.6317, -30.6106) (-114.6177, -30.5771) (-114.6038, -30.5434) (-114.5901, -30.5096) (-114.5765, -30.4756) (-114.5632, -30.4415) (-114.55, -30.4072) (-114.537, -30.3728) (-114.5242, -30.3383) (-114.5116, -30.3037) (-114.4991, -30.2689) (-114.4868, -30.234) (-114.4747, -30.199) (-114.4628, -30.1639) (-114.451, -30.1286) (-114.4394, -30.0932) (-114.4279, -30.0577) (-114.4167, -30.0221) (-114.4056, -29.9863) (-114.3946, -29.9505) (-114.3839, -29.9145) (-114.3733, -29.8784) (-114.3629, -29.8422) (-114.3526, -29.8059) (-114.3425, -29.7695) (-114.3326, -29.7329) (-114.3228, -29.6963) (-114.3132, -29.6596) (-114.3038, -29.6227) (-114.2946, -29.5858) (-114.2873, -29.5561) (-114.2819, -29.5338) (-114.2783, -29.519) (-114.2766, -29.5115) knots 0 0 0 0 0 0 0.01428571 0.02857143 0.04285714 0.05714286 0.07142857 0.08571429 0.1 0.11428571 0.12857143 0.14285714 0.15714286 0.17142857 0.18571429 0.2 0.21428571 0.22857143 0.24285714 0.25714286 0.27142857 0.28571429 0.3 0.31428571 0.32857143 0.34285714 0.35714286 0.37142857 0.38571429 0.4 0.41428571 0.42857143 0.44285714 0.45714286 0.47142857 0.48571429 0.5 0.51428571 0.52857143 0.54285714 0.55714286 0.57142857 0.58571429 0.6 0.61428571 0.62857143 0.64285714 0.65714286 0.67142857 0.68571429 0.7 0.71428571 0.72857143 0.74285714 0.75714286 0.77142857 0.78571429 0.8 0.81428571 0.82857143 0.84285714 0.85714286 0.87142857 0.88571429 0.9 0.91428571 0.92857143 0.94285714 0.95714286 0.97142857 0.98571429 1 1 1 1 1 1
  arc A25 (-114.2766, -29.5115) -> (-114.9538, -28.8611) centre (-125, -40) ccw
  spline S13 degree 5 poles (-117.1643, -30.0234) (-117.1601, -30.018) (-117.1516, -30.0075) (-117.1384, -29.992) (-117.12, -29.9721) (-117.0959, -29.9481) (-117.0709, -29.9248) (-117.0455, -29.902) (-117.0199, -29.8794) (-116.994, -29.8569) (-116.9679, -29.8346) (-116.9416, -29.8125) (-116.915, -29.7907) (-116.888, -29.7692) (-116.8606, -29.7481) (-116.8329, -29.7273) (-116.8048, -29.7068) (-116.7765, -29.6866) (-116.748, -29.6665) (-116.7193, -29.6466) (-116.6904, -29.6269) (-116.6613, -29.6075) (-116.632, -29.5882) (-116.6024, -29.5692) (-116.5726, -29.5504) (-116.5426, -29.5318) (-116.5124, -29.5134) (-116.4819, -29.4952) (-116.4513, -29.4772) (-116.4206, -29.4594) (-116.3896, -29.4418) (-116.3585, -29.4244) (-116.3271, -29.4072) (-116.2956, -29.3901) (-116.264, -29.3733) (-116.2321, -29.3566) (-116.2001, -29.3401) (-116.1679, -29.3238) (-116.1356, -29.3077) (-116.1031, -29.2918) (-116.0705, -29.276) (-116.0377, -29.2604) (-116.0047, -29.245) (-115.9716, -29.2298) (-115.9384, -29.2147) (-115.905, -29.1999) (-115.8714, -29.1851) (-115.8377, -29.1706) (-115.8039, -29.1562) (-115.7699, -29.142) (-115.7358, -29.128) (-115.7016, -29.1141) (-115.6672, -29.1004) (-115.6327, -29.0869) (-115.5981, -29.0735) (-115.5633, -29.0603) (-115.5284, -29.0473) (-115.4934, -29.0345) (-115.4583, -29.0218) (-115.423, -29.0092) (-115.3876, -28.9969) (-115.3521, -28.9847) (-115.3165, -28.9726) (-115.2807, -28.9607) (-115.2449, -28.949) (-115.2089, -28.9375) (-115.1728, -28.9261) (-115.1366, -28.9148) (-115.1003, -28.9038) (-115.0638, -28.8928) (-115.0273, -28.8821) (-114.998, -28.8736) (-114.9759, -28.8673) (-114.9612, -28.8632) (-114.9538, -28.8611) knots 0 0 0 0 0 0 0.01428571 0.02857143 0.04285714 0.05714286 0.07142857 0.08571429 0.1 0.11428571 0.12857143 0.14285714 0.15714286 0.17142857 0.18571429 0.2 0.21428571 0.22857143 0.24285714 0.25714286 0.27142857 0.28571429 0.3 0.31428571 0.32857143 0.34285714 0.35714286 0.37142857 0.38571429 0.4 0.41428571 0.42857143 0.44285714 0.45714286 0.47142857 0.48571429 0.5 0.51428571 0.52857143 0.54285714 0.55714286 0.57142857 0.58571429 0.6 0.61428571 0.62857143 0.64285714 0.65714286 0.67142857 0.68571429 0.7 0.71428571 0.72857143 0.74285714 0.75714286 0.77142857 0.78571429 0.8 0.81428571 0.82857143 0.84285714 0.85714286 0.87142857 0.88571429 0.9 0.91428571 0.92857143 0.94285714 0.95714286 0.97142857 0.98571429 1 1 1 1 1 1
  line L13 (-117.1643, -30.0234) -> (-117.4309, -30.3628)
  arc A26 (-118.1167, -30.4594) -> (-117.4309, -30.3628) centre (-117.8241, -30.0539) ccw
  arc A27 (-118.1167, -30.4594) -> (-118.788, -30.0093) centre (-125, -40) ccw
  arc A28 (-118.959, -29.3382) -> (-118.788, -30.0093) centre (-118.524, -29.5847) ccw
  line L14 (-118.959, -29.3382) -> (-118.7463, -28.9627)